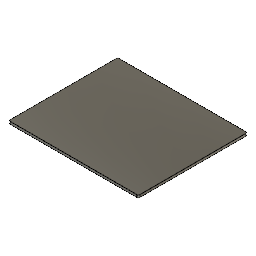
bear_full_surface_bed (Autodesk Fusion 360 design; units mm, degrees)
Autodesk Fusion 360 part; units mm, degrees
sketch "Sketch1" plane through (0, 0, 0) normal (0, 0, 1) x (1, 0, 0)
  line L0 (0, 0) -> (250, 0)
  line L1 (250, 0) -> (250, 210)
  line L2 (250, 210) -> (0, 210)
  line L3 (0, 210) -> (0, 0)
  dimension "d1" = 250
  dimension "d2" = 210
  constraint horizontal L0
  constraint vertical L1
  constraint horizontal L2
  constraint vertical L3
  constraint coincident L0.start L3.end
  measures "d1" distance of L0.start L0.end
  measures "d2" distance of L0.start L2.end
extrude "Extrude1" add sketch "Sketch1" along normal blind 5
fillet "Fillet1" radius 3 4 edges at (0, 0, 2.5) (0, 210, 2.5) (250, 210, 2.5) (250, 0, 2.5)
